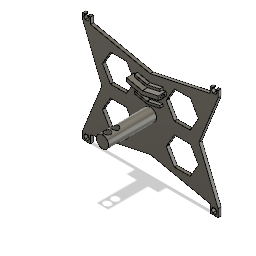
top (Autodesk Fusion 360 design; units mm, degrees)
Autodesk Fusion 360 part; units mm, degrees
sketch "Sketch1" plane through (0, 0, 0) normal (0, 0, 1) x (1, 0, 0)
  line L0 (0, 0) -> (105, 0) construction
  line L1 (105, 0) -> (105, 60) construction
  line L2 (105, 60) -> (0, 60) construction
  line L3 (0, 60) -> (0, 0) construction
  line L4 (15, 60) -> (52.5, 52)
  line L5 (52.5, 52) -> (90, 60)
  line L6 (90, 60) -> (90, 64)
  line L7 (95, -5) -> (90, -5)
  line L8 (90, -5) -> (90, 0)
  line L9 (90, 0) -> (52.5, 8)
  line L10 (52.5, 8) -> (15, 0)
  line L11 (15, 0) -> (15, -5)
  line L12 (15, -5) -> (10, -5)
  line L13 (15, 64) -> (15, 60)
  line L14 (95, 64) -> (95, 60)
  line L15 (95, 60) -> (83, 30)
  line L16 (83, 30) -> (95, 0)
  line L17 (95, 0) -> (95, -5)
  line L18 (10, 60) -> (22, 30)
  line L19 (22, 30) -> (10, 0)
  line L20 (10, -5) -> (10, 0)
  line L21 (52.5, 52) -> (52.5, 60) construction
  line L22 (95, 60) -> (95, 0) construction
  line L23 (83, 30) -> (95, 30) construction
  line L24 (10, 64) -> (10, 65) construction
  line L25 (10, 65) -> (15, 65) construction
  line L26 (15, 65) -> (15, 64) construction
  line L27 (90, 64) -> (90, 65) construction
  line L28 (90, 65) -> (95, 65) construction
  line L29 (95, 65) -> (95, 64) construction
  line L30 (12.5, 65) -> (12.5, 60) construction
  line L31 (92.5, 65) -> (92.5, 60) construction
  line L32 (52.5, 8) -> (52.5, 0) construction
  line L33 (10, 64) -> (10, 60)
  line L34 (14.2321, 62.5) -> (13.366, 64)
  line L35 (13.366, 64) -> (11.634, 64) construction
  line L36 (11.634, 64) -> (10.7679, 62.5)
  line L37 (10.7679, 62.5) -> (11.634, 61)
  line L38 (11.634, 61) -> (13.366, 61)
  line L39 (13.366, 61) -> (14.2321, 62.5)
  line L40 (11.634, 64) -> (10, 64)
  line L41 (94.2321, 62.5) -> (93.366, 64)
  line L42 (93.366, 64) -> (91.634, 64) construction
  line L43 (91.634, 64) -> (90.7679, 62.5)
  line L44 (90.7679, 62.5) -> (91.634, 61)
  line L45 (91.634, 61) -> (93.366, 61)
  line L46 (93.366, 61) -> (94.2321, 62.5)
  line L47 (13.366, 64) -> (15, 64)
  line L48 (90, 64) -> (91.634, 64)
  line L49 (93.366, 64) -> (95, 64)
  line L50 (12.5, -5) -> (12.5, 0) construction
  line L51 (92.5, -5) -> (92.5, 0) construction
  line L52 (94.2321, -2.5) -> (93.366, -1)
  line L53 (93.366, -1) -> (91.634, -1)
  line L54 (91.634, -1) -> (90.7679, -2.5)
  line L55 (90.7679, -2.5) -> (91.634, -4)
  line L56 (91.634, -4) -> (93.366, -4)
  line L57 (93.366, -4) -> (94.2321, -2.5)
  line L58 (14.2321, -2.5) -> (13.366, -1)
  line L59 (13.366, -1) -> (11.634, -1)
  line L60 (11.634, -1) -> (10.7679, -2.5)
  line L61 (10.7679, -2.5) -> (11.634, -4)
  line L62 (11.634, -4) -> (13.366, -4)
  line L63 (13.366, -4) -> (14.2321, -2.5)
  line L64 (52.5, 52) -> (52.5, 8) construction
  line L65 (72.5, 42.5) -> (32.5, 42.5) construction
  line L66 (32.5, 42.5) -> (32.5, 17.5) construction
  line L67 (32.5, 17.5) -> (72.5, 17.5) construction
  line L68 (72.5, 17.5) -> (72.5, 42.5) construction
  line L69 (72.5, 42.5) -> (32.5, 17.5) construction
  line L70 (32.5, 42.5) -> (72.5, 17.5) construction
  line L71 (27.5, 33.8397) -> (37.5, 33.8397)
  line L72 (37.5, 33.8397) -> (42.5, 42.5)
  line L73 (42.5, 42.5) -> (37.5, 51.1603)
  line L74 (37.5, 51.1603) -> (27.5, 51.1603)
  line L75 (27.5, 51.1603) -> (22.5, 42.5)
  line L76 (22.5, 42.5) -> (27.5, 33.8397)
  line L77 (77.5, 51.1603) -> (67.5, 51.1603)
  line L78 (67.5, 51.1603) -> (62.5, 42.5)
  line L79 (62.5, 42.5) -> (67.5, 33.8397)
  line L80 (67.5, 33.8397) -> (77.5, 33.8397)
  line L81 (77.5, 33.8397) -> (82.5, 42.5)
  line L82 (82.5, 42.5) -> (77.5, 51.1603)
  line L83 (77.5, 8.8397) -> (82.5, 17.5)
  line L84 (82.5, 17.5) -> (77.5, 26.1603)
  line L85 (77.5, 26.1603) -> (67.5, 26.1603)
  line L86 (67.5, 26.1603) -> (62.5, 17.5)
  line L87 (62.5, 17.5) -> (67.5, 8.8397)
  line L88 (67.5, 8.8397) -> (77.5, 8.8397)
  line L89 (27.5, 8.8397) -> (37.5, 8.8397)
  line L90 (37.5, 8.8397) -> (42.5, 17.5)
  line L91 (42.5, 17.5) -> (37.5, 26.1603)
  line L92 (37.5, 26.1603) -> (27.5, 26.1603)
  line L93 (27.5, 26.1603) -> (22.5, 17.5)
  line L94 (22.5, 17.5) -> (27.5, 8.8397)
  point P0 (12.5, 62.5)
  point P1 (92.5, 62.5)
  point P2 (92.5, -2.5)
  point P3 (12.5, -2.5)
  point P4 (52.5, 30)
  point P5 (32.5, 42.5)
  point P6 (72.5, 42.5)
  point P7 (72.5, 17.5)
  point P8 (32.5, 17.5)
  dimension "d1" = 105
  dimension "d2" = 60
  dimension "d3" = 5
  dimension "d4" = 5
  dimension "d5" = 10
  dimension "d9" = 8
  dimension "d10" = 12
  dimension "d11" = 5
  dimension "d12" = 5
  dimension "d13" = 1.5
  dimension "d45" = 40
  dimension "d46" = 25
  dimension "d47" = 10
  constraint horizontal L0
  constraint vertical L1
  constraint horizontal L2
  constraint vertical L3
  constraint coincident L0.start L3.end
  constraint coincident L2 L4.start
  constraint coincident L2 L5.end
  constraint perpendicular L2 L6
  constraint coincident L0 L8.end
  constraint perpendicular L0 L8
  constraint coincident L0 L10.end
  constraint perpendicular L0 L11
  constraint perpendicular L11 L12
  constraint perpendicular L2 L13
  constraint coincident L4.start L13.end
  constraint coincident L0 L16.end
  constraint perpendicular L0 L17
  constraint coincident L2 L18.start
  constraint coincident L0 L19.end
  constraint perpendicular L0 L20
  constraint equal L8 L11
  constraint equal L6 L13
  constraint horizontal L7
  constraint equal L7 L12
  constraint coincident L2 L14.end
  constraint equal L4 L5
  constraint equal L4 L10
  constraint equal L9 L10
  constraint equal L15 L16
  constraint equal L16 L18
  constraint equal L18 L19
  constraint midpoint L2 L21.end
  constraint midpoint L22 L23.end
  constraint perpendicular L24 L25
  constraint parallel L6 L27
  constraint perpendicular L27 L28
  constraint midpoint L25 L30.start
  constraint coincident L2 L30.end
  constraint perpendicular L2 L30
  constraint midpoint L28 L31.start
  constraint coincident L2 L31.end
  constraint perpendicular L2 L31
  constraint equal L25 L28
  constraint equal L7 L28
  constraint vertical L29
  constraint vertical L14
  constraint vertical L26
  constraint vertical L22
  constraint vertical L21
  constraint midpoint L0 L32.end
  constraint vertical L32
  constraint midpoint L30 P0
  constraint horizontal L35
  constraint vertical L33
  constraint vertical L24
  constraint horizontal L40
  constraint coincident L24.start L33.start
  constraint equal L6 L14
  constraint midpoint L31 P1
  constraint horizontal L42
  constraint equal L35 L42
  constraint coincident L26 L13.start
  constraint perpendicular L26 L47
  constraint coincident L13.start L26.end
  constraint midpoint L12 L50.start
  constraint coincident L0 L50.end
  constraint perpendicular L0 L50
  constraint midpoint L7 L51.start
  constraint coincident L0 L51.end
  constraint perpendicular L0 L51
  constraint midpoint L51 P2
  constraint midpoint L50 P3
  constraint horizontal L59
  constraint equal L53 L59
  constraint equal L38 L59
  constraint horizontal L53
  constraint perpendicular L65 L66
  constraint parallel L65 L67
  constraint parallel L66 L68
  constraint horizontal L65
  constraint coincident L69 P4
  constraint coincident L70 P4
  constraint midpoint L64 P4
  constraint coincident P5 L65.end
  constraint coincident P6 L65.start
  constraint coincident P7 L67.end
  constraint coincident P8 L66.end
  constraint horizontal L92
  constraint horizontal L74
  constraint horizontal L77
  constraint horizontal L85
  constraint equal L74 L77
  constraint equal L77 L85
  constraint equal L85 L92
  measures "d1" distance of L0.start L0.end
  measures "d2" distance of L0.start L2.end
  measures "d3" distance of L11.end L12.end
  measures "d4" distance of L12.end L19.end
  measures "d5" distance of L2.end L18.start
  measures "d9" distance of L4.end L21.end
  measures "d10" distance of L15.end L23.end
  measures "d11" distance of L18.start L24.end
  measures "d12" distance of L5.end L27.end
  measures "d13" distance of P0 L39
  measures "d45" distance of P6 P5
  measures "d46" distance of P6 P7
  measures "d47" distance of L73.end L74.end
extrude "Extrude1" add sketch "Sketch1" along normal blind 2 makes body 1
sketch "Sketch2" plane through (0, 0, 2) normal (0, 0, 1) x (1, 0, 0)
  line L0 (14.2321, -2.5) -> (13.366, -4)
  line L1 (13.366, -4) -> (11.634, -4)
  line L2 (11.634, -4) -> (10.7679, -2.5)
  line L3 (10.7679, -2.5) -> (11.634, -1)
  line L4 (11.634, -1) -> (13.366, -1)
  line L5 (13.366, -1) -> (14.2321, -2.5)
  line L6 (94.2321, -2.5) -> (93.366, -4)
  line L7 (93.366, -4) -> (91.634, -4)
  line L8 (91.634, -4) -> (90.7679, -2.5)
  line L9 (90.7679, -2.5) -> (91.634, -1)
  line L10 (91.634, -1) -> (93.366, -1)
  line L11 (93.366, -1) -> (94.2321, -2.5)
  line L12 (11.634, 64) -> (10, 64)
  line L13 (10, 64) -> (10, 60)
  line L14 (10, 60) -> (22, 30)
  line L15 (22, 30) -> (10, 0)
  line L16 (10, 0) -> (10, -5)
  line L17 (10, -5) -> (15, -5)
  line L18 (15, -5) -> (15, 0)
  line L19 (15, 0) -> (52.5, 8)
  line L20 (52.5, 8) -> (90, 0)
  line L21 (90, 0) -> (90, -5)
  line L22 (90, -5) -> (95, -5)
  line L23 (95, -5) -> (95, 0)
  line L24 (95, 0) -> (83, 30)
  line L25 (83, 30) -> (95, 60)
  line L26 (95, 60) -> (95, 64)
  line L27 (95, 64) -> (93.366, 64)
  line L28 (93.366, 64) -> (94.2321, 62.5)
  line L29 (94.2321, 62.5) -> (93.366, 61)
  line L30 (93.366, 61) -> (91.634, 61)
  line L31 (91.634, 61) -> (90.7679, 62.5)
  line L32 (90.7679, 62.5) -> (91.634, 64)
  line L33 (91.634, 64) -> (90, 64)
  line L34 (90, 64) -> (90, 60)
  line L35 (90, 60) -> (52.5, 52)
  line L36 (52.5, 52) -> (15, 60)
  line L37 (15, 60) -> (15, 64)
  line L38 (15, 64) -> (13.366, 64)
  line L39 (13.366, 64) -> (14.2321, 62.5)
  line L40 (14.2321, 62.5) -> (13.366, 61)
  line L41 (13.366, 61) -> (11.634, 61)
  line L42 (11.634, 61) -> (10.7679, 62.5)
  line L43 (10.7679, 62.5) -> (11.634, 64)
  line L44 (52.5, 52) -> (44.5, 53.7067) construction
  line L45 (44.5, 48.7067) -> (52.5, 47)
  line L46 (52.5, 47) -> (60.5, 48.7067)
  line L47 (60.5, 48.7067) -> (60.5, 47.2067)
  line L48 (60.5, 47.2067) -> (52.5, 45.5)
  line L49 (52.5, 45.5) -> (44.5, 47.2067)
  line L50 (44.5, 47.2067) -> (44.5, 48.7067)
  line L51 (60.5, 48.7067) -> (60.5, 53.7067) construction
  line L52 (44.5, 48.7067) -> (44.5, 53.7067) construction
  line L53 (44.5, 47.2067) -> (44.5, 44.2067) construction
  line L54 (52.5, 45.5) -> (52.5, 42.5) construction
  line L55 (52.5, 42.5) -> (60.5, 44.2067)
  line L56 (60.5, 44.2067) -> (60.5, 47.2067) construction
  line L57 (44.5, 44.2067) -> (52.5, 42.5)
  line L58 (44.5, 44.2067) -> (44.5, 42.7067)
  line L59 (44.5, 42.7067) -> (52.5, 41)
  line L60 (52.5, 41) -> (60.5, 42.7067)
  line L61 (60.5, 42.7067) -> (60.5, 44.2067)
  line L62 (52.5, 42.5) -> (52.5, 41) construction
  line L63 (44.5, 42.7067) -> (44.5, 39.7067) construction
  line L64 (44.5, 39.7067) -> (52.5, 38)
  line L65 (52.5, 38) -> (60.5, 39.7067)
  line L66 (60.5, 39.7067) -> (60.5, 42.7067) construction
  line L67 (52.5, 41) -> (52.5, 38) construction
  line L68 (44.5, 39.7067) -> (44.5, 38.2067)
  line L69 (44.5, 38.2067) -> (52.5, 36.5)
  line L70 (52.5, 36.5) -> (60.5, 38.2067)
  line L71 (60.5, 38.2067) -> (60.5, 39.7067)
  line L72 (52.5, 38) -> (52.5, 36.5) construction
  line L73 (52.5, 45.5) -> (52.5, 47) construction
  line L74 (52.5, 52) -> (60.5, 53.7067) construction
  line L75 (52.5, 52) -> (52.5, 47) construction
  line L76 (27.5, 8.8397) -> (22.5, 17.5)
  line L77 (22.5, 17.5) -> (27.5, 26.1603)
  line L78 (27.5, 26.1603) -> (37.5, 26.1603)
  line L79 (37.5, 26.1603) -> (42.5, 17.5)
  line L80 (42.5, 17.5) -> (37.5, 8.8397)
  line L81 (37.5, 8.8397) -> (27.5, 8.8397)
  line L82 (77.5, 8.8397) -> (67.5, 8.8397)
  line L83 (67.5, 8.8397) -> (62.5, 17.5)
  line L84 (62.5, 17.5) -> (67.5, 26.1603)
  line L85 (67.5, 26.1603) -> (77.5, 26.1603)
  line L86 (77.5, 26.1603) -> (82.5, 17.5)
  line L87 (82.5, 17.5) -> (77.5, 8.8397)
  line L88 (27.5, 33.8397) -> (22.5, 42.5)
  line L89 (22.5, 42.5) -> (27.5, 51.1603)
  line L90 (27.5, 51.1603) -> (37.5, 51.1603)
  line L91 (37.5, 51.1603) -> (42.5, 42.5)
  line L92 (42.5, 42.5) -> (37.5, 33.8397)
  line L93 (37.5, 33.8397) -> (27.5, 33.8397)
  line L94 (77.5, 51.1603) -> (82.5, 42.5)
  line L95 (82.5, 42.5) -> (77.5, 33.8397)
  line L96 (77.5, 33.8397) -> (67.5, 33.8397)
  line L97 (67.5, 33.8397) -> (62.5, 42.5)
  line L98 (62.5, 42.5) -> (67.5, 51.1603)
  line L99 (67.5, 51.1603) -> (77.5, 51.1603)
  dimension "d16" = 5
  dimension "d17" = 3
  dimension "d18" = 1.5
  dimension "d19" = 8
  constraint coincident L35.end L36.start
  constraint coincident L36 L44.end
  constraint coincident L35 L51.end
  constraint vertical L54
  constraint vertical L56
  constraint vertical L61
  constraint vertical L66
  constraint vertical L71
  constraint vertical L62
  constraint vertical L75
  constraint vertical L73
  constraint vertical L67
  constraint vertical L72
  constraint vertical L52
  constraint vertical L51
  constraint vertical L47
  constraint vertical L50
  constraint vertical L53
  constraint vertical L58
  constraint vertical L63
  constraint vertical L68
  constraint equal L52 L75
  constraint equal L51 L75
  constraint equal L54 L56
  constraint equal L53 L54
  constraint equal L53 L63
  constraint equal L63 L67
  constraint equal L66 L67
  constraint equal L50 L73
  constraint equal L47 L73
  constraint equal L47 L61
  constraint equal L61 L62
  constraint equal L58 L62
  constraint equal L58 L68
  constraint equal L68 L72
  constraint equal L71 L72
  constraint equal L45 L46
  measures "d16" distance of L44.end L45.start
  measures "d17" distance of L49.end L53.end
  measures "d18" distance of L45.start L49.end
  measures "d19" horizontal distance of L45.start L45.end
extrude "Extrude2" add sketch "Sketch2" along normal blind 2 contours L45 L46 L47 L48 L49 L50 | L55 L57 L58 L59 L60 L61 | L64 L65 L68 L69 L70 L71 bodies 1
sketch "Sketch4" plane through (0, 0, 2) normal (0, 0, 1) x (1, 0, 0)
  line L0 (60.5, 38.2067) -> (52.5, 36.5)
  line L1 (52.5, 36.5) -> (44.5, 38.2067)
  line L2 (44.5, 44.2067) -> (52.5, 42.5)
  line L3 (52.5, 42.5) -> (60.5, 44.2067)
  line L4 (44.5, 47.2067) -> (44.5, 48.7067)
  line L5 (44.5, 48.7067) -> (52.5, 47)
  line L6 (52.5, 47) -> (60.5, 48.7067)
  line L7 (60.5, 48.7067) -> (60.5, 47.2067)
  line L8 (60.5, 47.2067) -> (52.5, 45.5)
  line L9 (52.5, 45.5) -> (44.5, 47.2067)
  line L10 (14.2321, -2.5) -> (13.366, -4)
  line L11 (13.366, -4) -> (11.634, -4)
  line L12 (11.634, -4) -> (10.7679, -2.5)
  line L13 (10.7679, -2.5) -> (11.634, -1)
  line L14 (11.634, -1) -> (13.366, -1)
  line L15 (13.366, -1) -> (14.2321, -2.5)
  line L16 (94.2321, -2.5) -> (93.366, -4)
  line L17 (93.366, -4) -> (91.634, -4)
  line L18 (91.634, -4) -> (90.7679, -2.5)
  line L19 (90.7679, -2.5) -> (91.634, -1)
  line L20 (91.634, -1) -> (93.366, -1)
  line L21 (93.366, -1) -> (94.2321, -2.5)
  line L22 (11.634, 64) -> (10, 64)
  line L23 (10, 64) -> (10, 60)
  line L24 (10, 60) -> (22, 30)
  line L25 (22, 30) -> (10, 0)
  line L26 (10, 0) -> (10, -5)
  line L27 (10, -5) -> (15, -5)
  line L28 (15, -5) -> (15, 0)
  line L29 (15, 0) -> (52.5, 8)
  line L30 (52.5, 8) -> (90, 0)
  line L31 (90, 0) -> (90, -5)
  line L32 (90, -5) -> (95, -5)
  line L33 (95, -5) -> (95, 0)
  line L34 (95, 0) -> (83, 30)
  line L35 (83, 30) -> (95, 60)
  line L36 (95, 60) -> (95, 64)
  line L37 (95, 64) -> (93.366, 64)
  line L38 (93.366, 64) -> (94.2321, 62.5)
  line L39 (94.2321, 62.5) -> (93.366, 61)
  line L40 (93.366, 61) -> (91.634, 61)
  line L41 (91.634, 61) -> (90.7679, 62.5)
  line L42 (90.7679, 62.5) -> (91.634, 64)
  line L43 (91.634, 64) -> (90, 64)
  line L44 (90, 64) -> (90, 60)
  line L45 (90, 60) -> (52.5, 52)
  line L46 (52.5, 52) -> (15, 60)
  line L47 (15, 60) -> (15, 64)
  line L48 (15, 64) -> (13.366, 64)
  line L49 (13.366, 64) -> (14.2321, 62.5)
  line L50 (14.2321, 62.5) -> (13.366, 61)
  line L51 (13.366, 61) -> (11.634, 61)
  line L52 (11.634, 61) -> (10.7679, 62.5)
  line L53 (10.7679, 62.5) -> (11.634, 64)
  line L54 (22, 30) -> (83, 30) construction
  circle A0 centre (52.5, 30) radius 3.9
  line L55 (42.5, 42.5) -> (37.5, 33.8397)
  line L56 (37.5, 33.8397) -> (27.5, 33.8397)
  line L57 (27.5, 33.8397) -> (22.5, 42.5)
  line L58 (22.5, 42.5) -> (27.5, 51.1603)
  line L59 (27.5, 51.1603) -> (37.5, 51.1603)
  line L60 (37.5, 51.1603) -> (42.5, 42.5)
  line L61 (62.5, 42.5) -> (67.5, 51.1603)
  line L62 (67.5, 51.1603) -> (77.5, 51.1603)
  line L63 (77.5, 51.1603) -> (82.5, 42.5)
  line L64 (82.5, 42.5) -> (77.5, 33.8397)
  line L65 (77.5, 33.8397) -> (67.5, 33.8397)
  line L66 (67.5, 33.8397) -> (62.5, 42.5)
  line L67 (77.5, 8.8397) -> (67.5, 8.8397)
  line L68 (67.5, 8.8397) -> (62.5, 17.5)
  line L69 (62.5, 17.5) -> (67.5, 26.1603)
  line L70 (67.5, 26.1603) -> (77.5, 26.1603)
  line L71 (77.5, 26.1603) -> (82.5, 17.5)
  line L72 (82.5, 17.5) -> (77.5, 8.8397)
  line L73 (27.5, 8.8397) -> (22.5, 17.5)
  line L74 (22.5, 17.5) -> (27.5, 26.1603)
  line L75 (27.5, 26.1603) -> (37.5, 26.1603)
  line L76 (37.5, 26.1603) -> (42.5, 17.5)
  line L77 (42.5, 17.5) -> (37.5, 8.8397)
  line L78 (37.5, 8.8397) -> (27.5, 8.8397)
  line L79 (44.5, 39.7067) -> (52.5, 38)
  line L80 (52.5, 38) -> (60.5, 39.7067)
  line L81 (60.5, 39.7067) -> (60.5, 38.2067)
  line L82 (44.5, 38.2067) -> (44.5, 39.7067)
  line L83 (60.5, 42.7067) -> (52.5, 41)
  line L84 (52.5, 41) -> (44.5, 42.7067)
  line L85 (60.5, 44.2067) -> (60.5, 42.7067)
  line L86 (44.5, 42.7067) -> (44.5, 44.2067)
  dimension "d24" = 7.8
  constraint coincident L24.end L25.start
  constraint coincident L34.end L35.start
  constraint midpoint L54 A0.centre
  measures "d24" diameter of A0
extrude "Extrude3" add sketch "Sketch4" along normal blind 30 contours A0 bodies 1
sketch "Sketch5" plane through (0, 0, 0) normal (0, 1, 0) x (1, 0, 0)
  line L0 (0, 0) -> (52.5, 0) construction
  line L1 (52.5, 0) -> (52.5, -24) construction
  line L2 (52.5, -24) -> (52.5, -29) construction
  circle A0 centre (52.5, -29) radius 2
  circle A1 centre (52.5, -24) radius 2
  dimension "d27" = 52.5
  dimension "d28" = 5
  dimension "d29" = 24
  dimension "d30" = 4
  dimension "d31" = 4
  constraint coincident L0.start origin
  constraint horizontal L0
  constraint perpendicular L0 L1
  constraint parallel L1 L2
  constraint coincident L2.end A0.centre
  constraint coincident L1.end L2.start
  measures "d27" distance of L0.start L0.end
  measures "d28" distance of L1.end L2.end
  measures "d29" distance of L0.end L1.end
  measures "d30" diameter of A0
  measures "d31" diameter of A1
extrude "Extrude4" cut sketch "Sketch5" along normal through all bodies 1
sketch "Sketch9" plane through (0, 0, 2) normal (0, 0, 1) x (1, 0, 0)
  circle A0 centre (52.5, 30) radius 3.9
  line L0 (44.5, 39.7067) -> (52.5, 38)
  line L1 (52.5, 38) -> (60.5, 39.7067)
  line L2 (60.5, 39.7067) -> (60.5, 38.2067)
  line L3 (60.5, 38.2067) -> (52.5, 36.5)
  line L4 (52.5, 36.5) -> (44.5, 38.2067)
  line L5 (44.5, 38.2067) -> (44.5, 39.7067)
  line L6 (44.5, 44.2067) -> (52.5, 42.5)
  line L7 (52.5, 42.5) -> (60.5, 44.2067)
  line L8 (60.5, 44.2067) -> (60.5, 42.7067)
  line L9 (60.5, 42.7067) -> (52.5, 41)
  line L10 (52.5, 41) -> (44.5, 42.7067)
  line L11 (44.5, 42.7067) -> (44.5, 44.2067)
  line L12 (44.5, 47.2067) -> (44.5, 48.7067)
  line L13 (44.5, 48.7067) -> (52.5, 47)
  line L14 (52.5, 47) -> (60.5, 48.7067)
  line L15 (60.5, 48.7067) -> (60.5, 47.2067)
  line L16 (60.5, 47.2067) -> (52.5, 45.5)
  line L17 (52.5, 45.5) -> (44.5, 47.2067)
  line L18 (77.5, 51.1603) -> (82.5, 42.5)
  line L19 (82.5, 42.5) -> (77.5, 33.8397)
  line L20 (77.5, 33.8397) -> (67.5, 33.8397)
  line L21 (67.5, 33.8397) -> (62.5, 42.5)
  line L22 (62.5, 42.5) -> (67.5, 51.1603)
  line L23 (67.5, 51.1603) -> (77.5, 51.1603)
  line L24 (27.5, 8.8397) -> (22.5, 17.5)
  line L25 (22.5, 17.5) -> (27.5, 26.1603)
  line L26 (27.5, 26.1603) -> (37.5, 26.1603)
  line L27 (37.5, 26.1603) -> (42.5, 17.5)
  line L28 (42.5, 17.5) -> (37.5, 8.8397)
  line L29 (37.5, 8.8397) -> (27.5, 8.8397)
  line L30 (27.5, 33.8397) -> (22.5, 42.5)
  line L31 (22.5, 42.5) -> (27.5, 51.1603)
  line L32 (27.5, 51.1603) -> (37.5, 51.1603)
  line L33 (37.5, 51.1603) -> (42.5, 42.5)
  line L34 (42.5, 42.5) -> (37.5, 33.8397)
  line L35 (37.5, 33.8397) -> (27.5, 33.8397)
  line L36 (77.5, 8.8397) -> (67.5, 8.8397)
  line L37 (67.5, 8.8397) -> (62.5, 17.5)
  line L38 (62.5, 17.5) -> (67.5, 26.1603)
  line L39 (67.5, 26.1603) -> (77.5, 26.1603)
  line L40 (77.5, 26.1603) -> (82.5, 17.5)
  line L41 (82.5, 17.5) -> (77.5, 8.8397)
  line L42 (14.2321, -2.5) -> (13.366, -4)
  line L43 (13.366, -4) -> (11.634, -4)
  line L44 (11.634, -4) -> (10.7679, -2.5)
  line L45 (10.7679, -2.5) -> (11.634, -1)
  line L46 (11.634, -1) -> (13.366, -1)
  line L47 (13.366, -1) -> (14.2321, -2.5)
  line L48 (94.2321, -2.5) -> (93.366, -4)
  line L49 (93.366, -4) -> (91.634, -4)
  line L50 (91.634, -4) -> (90.7679, -2.5)
  line L51 (90.7679, -2.5) -> (91.634, -1)
  line L52 (91.634, -1) -> (93.366, -1)
  line L53 (93.366, -1) -> (94.2321, -2.5)
  line L54 (11.634, 64) -> (10, 64)
  line L55 (10, 64) -> (10, 60)
  line L56 (10, 60) -> (22, 30)
  line L57 (22, 30) -> (10, 0)
  line L58 (10, 0) -> (10, -5)
  line L59 (10, -5) -> (15, -5)
  line L60 (15, -5) -> (15, 0)
  line L61 (15, 0) -> (52.5, 8)
  line L62 (52.5, 8) -> (90, 0)
  line L63 (90, 0) -> (90, -5)
  line L64 (90, -5) -> (95, -5)
  line L65 (95, -5) -> (95, 0)
  line L66 (95, 0) -> (83, 30)
  line L67 (83, 30) -> (95, 60)
  line L68 (95, 60) -> (95, 64)
  line L69 (95, 64) -> (93.366, 64)
  line L70 (93.366, 64) -> (94.2321, 62.5)
  line L71 (94.2321, 62.5) -> (93.366, 61)
  line L72 (93.366, 61) -> (91.634, 61)
  line L73 (91.634, 61) -> (90.7679, 62.5)
  line L74 (90.7679, 62.5) -> (91.634, 64)
  line L75 (91.634, 64) -> (90, 64)
  line L76 (90, 64) -> (90, 60)
  line L77 (90, 60) -> (52.5, 52)
  line L78 (52.5, 52) -> (15, 60)
  line L79 (15, 60) -> (15, 64)
  line L80 (15, 64) -> (13.366, 64)
  line L81 (13.366, 64) -> (14.2321, 62.5)
  line L82 (14.2321, 62.5) -> (13.366, 61)
  line L83 (13.366, 61) -> (11.634, 61)
  line L84 (11.634, 61) -> (10.7679, 62.5)
  line L85 (10.7679, 62.5) -> (11.634, 64)
  line L86 (42.5, 47.3833) -> (42.5, 44.8833)
  line L87 (42.5, 44.8833) -> (52.5, 42.75)
  line L88 (52.5, 42.75) -> (62.5, 44.8833)
  line L89 (62.5, 44.8833) -> (62.5, 47.3833)
  line L90 (62.5, 47.3833) -> (52.5, 45.25)
  line L91 (52.5, 45.25) -> (42.5, 47.3833)
  line L92 (52.5, 45.5) -> (52.5, 45.25) construction
  line L93 (52.5, 42.75) -> (52.5, 42.5) construction
  line L94 (52.5, 42.75) -> (52.5, 45.25) construction
  dimension "d48" = 2.5
  dimension "d49" = 10
  constraint parallel L6 L87
  constraint parallel L7 L88
  constraint coincident L16.end L17.start
  constraint coincident L6.end L7.start
  constraint vertical L94
  constraint vertical L92
  constraint equal L86 L94
  constraint equal L89 L94
  constraint vertical L89
  constraint vertical L86
  constraint equal L92 L93
  constraint equal L90 L91
  measures "d48" distance of L86.start L86.end
  measures "d49" horizontal distance of L89.end L90.end
extrude "Extrude8" add sketch "Sketch9" along normal blind 5 separate body contours L86 L87 L88 L89 L90 L91 makes body 2
sketch "Sketch11" plane through (0, 0, 7) normal (0, 0, 1) x (1, 0, 0)
  line L0 (52.5, 45.25) -> (42.5, 47.3833)
  line L1 (42.5, 47.3833) -> (42.5, 44.8833)
  line L2 (42.5, 44.8833) -> (52.5, 42.75)
  line L3 (52.5, 42.75) -> (62.5, 44.8833)
  line L4 (62.5, 44.8833) -> (62.5, 47.3833)
  line L5 (62.5, 47.3833) -> (52.5, 45.25)
  line L6 (42.5, 46.5833) -> (52.5, 44.45)
  line L7 (52.5, 44.45) -> (62.5, 46.5833)
  line L8 (62.5, 45.6833) -> (62.5, 46.5833)
  line L9 (62.5, 45.6833) -> (52.5, 43.55)
  line L10 (52.5, 43.55) -> (42.5, 45.6833)
  dimension "d54" = 0.8
  dimension "d55" = 0.8
  dimension "d56" = 0.8
  dimension "d57" = 0.8
  constraint coincident L1 L6.start
  constraint coincident L4 L7.end
  constraint coincident L4 L8.start
  constraint parallel L7 L9
  constraint coincident L1 L10.end
  constraint parallel L5 L7
  constraint parallel L0 L6
  constraint parallel L6 L10
  measures "d54" distance of L4.end L7.end
  measures "d55" distance of L3.end L8.start
  measures "d56" distance of L0.end L6.start
  measures "d57" distance of L1.end L10.end
extrude "Extrude9" cut sketch "Sketch11" against normal up to surface (3 mm away) from surface at -1 contours L1 L4 L6 L7 L8 L9 L10 bodies 2
equation "d11 = d4"
equation "d12 = d11"
equation "d55 = d54"
equation "d56 = d54"
equation "d57 = d54"
